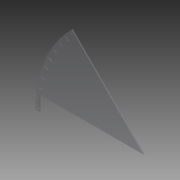
# Autodesk Inventor part: Side Panel 2
Saved by Autodesk Inventor 2013 (Build 170138000, 138)
## iProperties
Created: 2013-01-27
Part Number: Side Panel 2
Material: Polycarbonate, Clear
Document SubType Name: Modeling
Designer: Andrew Toennies
Density: 1.2 g/cm^3
Mass: 103.35 g
Surface Area: 573.396 cm^2
Volume: 86.1254 cm^3
Author: Andrew Toennies
Autodesk Inventor part; units mm, degrees
ref_plane "YZ Plane" through (0, 0, 0) normal (1, 0, 0) x (0, 1, 0)
ref_plane "XZ Plane" through (0, 0, 0) normal (0, 1, 0) x (-1, 0, 0)
ref_plane "XY Plane" through (0, 0, 0) normal (0, 0, 1) x (1, 0, 0)
sketch "Sketch3" plane through (0, 0, 0) normal (0, 0, 1) x (1, 0, 0)
  line L0 (-311.15, 0) -> (0, 0)
  line L1 (0, 0) -> (-220.0163, 220.0163)
  line L2 (-301.625, 0) -> (-301.625, 38.1)
  line L3 (-301.625, 38.1) -> (-38.1, 38.1)
  line L4 (-23.0461, 23.0461) -> (-23.0461, 0)
  circle A0 centre (0, 0) radius 311.15
  point P0 (0, 0)
  point P1 (-306.9751, 50.8)
  dimension "d10" = 38.1
  dimension "d12" = 9.525
  constraints: 10 end point, 4 point on line, 3 perpendicular, 3 point on circle, 1 centre point, 1 coincident, 1 horizontal, 5 other
  measures "d10" distance of L2.start L2.end
  measures "d12" distance of L0.start L2.start
extrude "Extrusion3" add sketch "Sketch3" along normal blind 3.175 contours A0 L1 L3 L2 L0
sketch "Sketch4" plane through (0, 0, 0) normal (0, 0, -1) x (-1, 0, 0)
  line L0 (-141.2846, 157.1654) -> (-0.3893, 16.2701) projected
  line L1 (-145.7747, 152.6753) -> (-141.2846, 157.1654) projected
  line L2 (-4.8794, 11.78) -> (-145.7747, 152.6753) projected
  arc A0 (0, 0) -> (-4.8794, 11.78) centre (-16.6594, 0) ccw projected
  line L3 (0, -6.35) -> (0, 0) projected
  line L4 (6.35, -6.35) -> (0, -6.35) projected
  line L5 (6.35, -2.6303) -> (6.35, -6.35) projected
  arc A1 (5.6464, 5.6464) -> (-0.3893, 16.2701) centre (-16.6594, 0) ccw projected
  line L6 (6.35, -2.6303) -> (214.3556, 205.3753) projected
  line L7 (209.9135, 209.9135) -> (5.6464, 5.6464) projected
  arc A2 (214.3556, 205.3753) -> (209.9135, 209.9135) centre (0, 0) ccw projected
  circle A3 centre (245.7763, 172.0944) radius 1.5875 projected
  circle A4 centre (271.9263, 126.8013) radius 1.5875 projected
  circle A5 centre (289.814, 77.6554) radius 1.5875 projected
  circle A6 centre (298.8958, 26.15) radius 1.5875 projected
  circle A7 centre (304.7338, 6.35) radius 1.5875 projected
  circle A8 centre (249.6775, 174.8261) radius 1.5875 projected
  circle A9 centre (276.2426, 128.814) radius 1.5875 projected
  circle A10 centre (294.4142, 78.888) radius 1.5875 projected
  circle A11 centre (303.6401, 26.5651) radius 1.5875 projected
  circle A12 centre (300.1694, 52.928) radius 1.5875 projected
  circle A13 centre (286.4183, 104.2477) radius 1.5875 projected
  circle A14 centre (263.9645, 152.4) radius 1.5875 projected
  circle A15 centre (233.4903, 195.9217) radius 1.5875 projected
  circle A16 centre (219.9695, 210.9892) radius 1.5875 projected
  circle A17 centre (295.4793, 52.101) radius 1.5875 projected
  circle A18 centre (281.943, 102.6189) radius 1.5875 projected
  circle A19 centre (259.8401, 150.0188) radius 1.5875 projected
  circle A20 centre (229.8421, 192.8604) radius 1.5875 projected
  arc A21 (311.15, 0) -> (220.0163, 220.0163) centre (0, 0) ccw projected
  line L8 (220.0163, 220.0163) -> (0, 0) projected
  line L9 (0, 0) -> (311.15, 0) projected
  point P0 (-16.6594, 0)
  point P1 (-16.6594, 0)
  point P2 (0, 0)
extrude "Extrusion5" cut sketch "Sketch4" against normal through all contours A3 | A4 | A5 | A7 | A8 | A9 | A10 | A12 | A13 | A14 | A15 | A16 | A17 | A18 | A19 | A20
body "Solid2"
